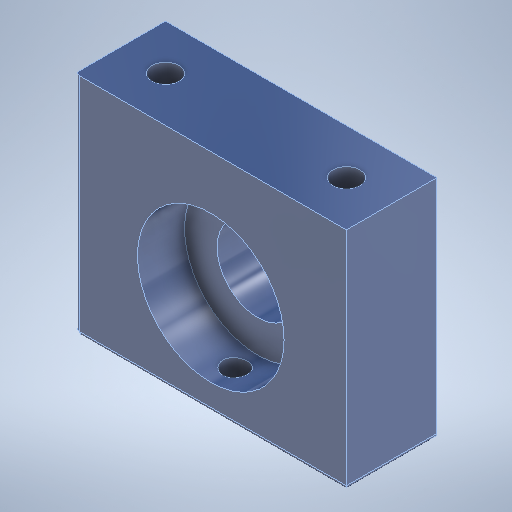
# Autodesk Inventor part: wheel_holder
Saved by Autodesk Inventor 2025 (Build 290162000, 162)
## iProperties
Created: 2024-06-27
Part Number: wheel_holder
Material: Generic
Document SubType Name: Modeling
Designer: Pintu
Density: 1 g/cm^3
Appearance: Flaked Satin - Blue
Author: Pintu
Autodesk Inventor part; units mm, degrees
ref_plane "YZ Plane" through (0, 0, 0) normal (1, 0, 0) x (0, 1, 0)
ref_plane "XZ Plane" through (0, 0, 0) normal (0, 1, 0) x (-1, 0, 0)
ref_plane "XY Plane" through (0, 0, 0) normal (0, 0, 1) x (1, 0, 0)
sketch "Sketch1" plane through (0, 0, 0) normal (0, 0, 1) x (1, 0, 0)
  line L0 (-15, 12.5) -> (15, 12.5)
  line L1 (15, 12.5) -> (15, -12.5)
  line L2 (15, -12.5) -> (-15, -12.5)
  line L3 (-15, -12.5) -> (-15, 12.5)
  line L4 (-15, 12.5) -> (15, -12.5) construction
  line L5 (15, 12.5) -> (-15, -12.5) construction
  point P0 (0, 0)
  dimension "d7" = 9
  dimension "d15" = 5
  dimension "d0" = 30
  dimension "d10" = 25
  constraints: 12 end point, 2 midpoint, 2 parallel, 1 horizontal, 1 perpendicular
  measures "d0" distance of L1.end L2.end
  measures "d10" distance of L0.end L1.end
extrude "Extrusion1" add sketch "Sketch1" along normal blind 10
sketch "Sketch2" plane through (0, 0, 10) normal (0, 0, 1) x (1, 0, 0)
  circle A0 centre (0, -1.5) radius 8.1
  line L0 (15, 12.5) -> (-15, 12.5) projected
  point P0 (0, 12.5)
  dimension "d4" = 16.2
  dimension "d38" = 14
  constraints: 1 centre point, 1 coincident, 1 midpoint
  measures "d4" diameter of A0
  measures "d38" distance of point (0, 12.5) point (0, -1.5)
extrude "Extrusion2" cut sketch "Sketch2" against normal blind 5.2
sketch "Sketch3" plane through (0, -1.5, 4.8) normal (0, 0, 1) x (1, 0, 0)
  circle A0 centre (0, 0) radius 4.5
  circle A1 centre (0, 0) radius 8.1 projected
  dimension "d7" = 9
  constraints: 1 centre point, 1 coincident, 1 concentric
  measures "d7" diameter of A0
extrude "Extrusion3" cut sketch "Sketch3" against normal blind 5.2 contours A0
sketch "Sketch4" plane through (-15, -12.5, 0) normal (0, -1, 0) x (1, 0, 0)
  line L0 (0, 0) -> (0, 10) projected
  line L1 (0, 10) -> (30, 10) projected
  point P0 (15, 0)
  point P1 (5, 5)
  dimension "d11" = 5
  dimension "d12" = 5
  measures "d11" distance from line of L0 point (5, 5)
  measures "d12" distance from line of L1 point (5, 5)
hole "Hole1" at (-10, -12.5, 5) direction (0, 1, 0) diameter 3 end through all counterbore diameter 5 counterbore depth 2
sketch "Sketch5" plane through (-15, -12.5, 0) normal (0, -1, 0) x (1, 0, 0)
  line L0 (30, 0) -> (30, 10) projected
  line L1 (0, 10) -> (30, 10) projected
  point P0 (15, 0)
  point P1 (25, 5)
  dimension "d20" = 5
  dimension "d21" = 5
  measures "d20" distance from line of L0 point (25, 5)
  measures "d21" distance from line of L1 point (25, 5)
hole "Hole2" at (10, -12.5, 5) direction (0, 1, 0) diameter 3 end through all counterbore diameter 5 counterbore depth 2
sketch "Sketch6" plane through (-15, -12.5, 0) normal (0, -1, 0) x (1, 0, 0)
  line L0 (0, 10) -> (30, 10) projected
  line L1 (30, 0) -> (30, 10) projected
  point P0 (15, 0)
  point P1 (15, 7.3)
  dimension "d29" = 2.7
  dimension "d30" = 15
  measures "d29" distance from line of L0 point (15, 7.3)
  measures "d30" distance from line of L1 point (15, 7.3)
hole "Hole3" at (0, -12.5, 7.3) direction (0, 1, 0) diameter 2.7 depth 8 tip angle 118
fillet "Fillet2" radius 0.5 5 edges at (-15, 0, 10) (0, -12.5, 0) (15, -12.5, 5) (-15, -12.5, 5) (0, -12.5, 10)
body "Solid1"
